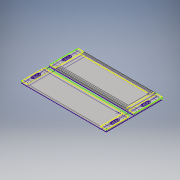
# Autodesk Inventor part: Fixture Base
Saved by Autodesk Inventor 2016 (Build 200138000, 138)
## iProperties
Created: 2016-04-07
Part Number: Fixture Base
Material: Generic
Document SubType Name: Modeling
Designer: Sam Clay
Density: 1 g/cm^3
Appearance: Default
Author: Sam Clay
Autodesk Inventor part; units mm, degrees
ref_plane "YZ Plane" through (0, 0, 0) normal (1, 0, 0) x (0, 1, 0)
ref_plane "XZ Plane" through (0, 0, 0) normal (0, 1, 0) x (-1, 0, 0)
ref_plane "XY Plane" through (0, 0, 0) normal (0, 0, 1) x (1, 0, 0)
sketch "Base Sketch" plane through (0, 0, 0) normal (0, 1, 0) x (-1, 0, 0)
  line L0 (0, 0) -> (660.4, 0)
  line L1 (660.4, 0) -> (660.4, 254)
  line L2 (660.4, 508) -> (0, 508)
  line L3 (0, 508) -> (0, 304.8)
  line L4 (0, 508) -> (-50.8, 508)
  line L5 (-50.8, 508) -> (-50.8, 304.8)
  line L6 (-50.8, 0) -> (0, 0)
  line L7 (0, 0) -> (0, 254)
  line L8 (660.4, 508) -> (711.2, 508)
  line L9 (711.2, 508) -> (711.2, 304.8)
  line L10 (711.2, 0) -> (660.4, 0)
  line L11 (660.4, 0) -> (660.4, 254)
  line L12 (660.4, 254) -> (660.4, 304.8)
  line L13 (711.2, 254) -> (711.2, 0)
  line L14 (0, 254) -> (0, 254)
  line L15 (-50.8, 254) -> (-50.8, 0)
  line L16 (711.2, 254) -> (660.4, 254)
  line L17 (711.2, 304.8) -> (660.4, 304.8)
  line L18 (711.2, 304.8) -> (711.2, 254)
  line L19 (711.2, 254) -> (711.2, 254)
  line L20 (660.4, 254) -> (660.4, 304.8)
  line L21 (660.4, 304.8) -> (660.4, 508)
  line L22 (0, 304.8) -> (0, 254)
  line L23 (0, 254) -> (0, 304.8)
  line L24 (-50.8, 254) -> (-50.8, 254)
  line L25 (-50.8, 304.8) -> (-50.8, 254)
  line L26 (660.4, 254) -> (0, 254)
  line L27 (660.4, 304.8) -> (0, 304.8)
  line L28 (0, 304.8) -> (-50.8, 304.8)
  line L29 (0, 254) -> (-50.8, 254)
  line L30 (0, 304.8) -> (0, 508)
  line L31 (0, 254) -> (0, 0)
  line L32 (660.4, 254) -> (660.4, 304.8)
  line L33 (660.4, 304.8) -> (660.4, 508)
  line L34 (635, 0) -> (635, 254)
  line L35 (25.4, 0) -> (25.4, 254)
  point P0 (660.4, 304.8)
  point P1 (660.4, 254)
  point P2 (660.4, 304.8)
  dimension "d0" = 660.4
  dimension "d87" = 50.8
  dimension "d88" = 50.8
  dimension "d165" = 254
  dimension "d166" = 50.8
  dimension "d167" = 203.2
  dimension "d172" = 25.4
  dimension "d173" = 25.4
  constraints: 72 end point, 43 parallel, 32 perpendicular, 14 coincident, 9 point on line, 3 horizontal
  measures "d0" distance of L2.end L2.start
  measures "d87" distance of L6.end L6.start
  measures "d88" distance of L10.start L10.end
  measures "d165" distance between parallel lines of L16 L0
  measures "d166" distance between parallel lines of L16 L17
  measures "d167" distance between parallel lines of L2 L17
  measures "d172" distance between parallel lines of L34 L1
  measures "d173" distance between parallel lines of L31 L35
extrude "Lower Level" add sketch "Base Sketch" along normal blind 17.78 contours L6 L15 L29 L7 | L28 L5 L4 L3 | L1 L16 L13 L10 | L21 L8 L9 L17
extrude "Base" add sketch "Base Sketch" along normal blind 19.05 contours L7 L26 L35 L0 | L35 L26 L34 L0 | L34 L26 L1 L0 | L3 L2 L21 L27
sketch "Tracks Sketch" plane through (0, 19.05, 0) normal (0, 1, 0) x (1, 0, 0)
  line L0 (-660.4, 0) -> (-660.4, -254) projected
  line L1 (0, -254) -> (0, 0) projected
  line L2 (-660.4, -22.987) -> (0, -22.987)
  line L3 (-660.4, -3.175) -> (0, -3.175)
  line L4 (-660.4, -231.013) -> (0, -231.013)
  line L5 (-660.4, -250.825) -> (0, -250.825)
  line L6 (-38.1, -35.687) -> (-660.4, -35.687)
  line L7 (-660.4, -35.687) -> (-660.4, -218.313)
  line L8 (-660.4, -218.313) -> (-38.1, -218.313)
  line L9 (-38.1, -218.313) -> (-38.1, -35.687)
  circle A0 centre (-41.91, -39.497) radius 8.89
  line L10 (-711.2, 0) -> (-711.2, -254) projected
  line L11 (50.8, -508) -> (50.8, -304.8) projected
  line L12 (-711.2, -508) -> (50.8, -508) projected
  line L13 (50.8, -304.8) -> (-711.2, -304.8) projected
  line L14 (-711.2, -254) -> (50.8, -254) projected
  line L15 (50.8, 0) -> (-711.2, 0) projected
  line L16 (-711.2, -304.8) -> (-711.2, -508) projected
  line L17 (50.8, -254) -> (50.8, 0) projected
  dimension "d170" = 19.812
  dimension "d171" = 19.812
  dimension "d174" = 38.1
  dimension "d175" = 12.7
  dimension "d176" = 12.7
  dimension "d177" = 182.626
  dimension "d178" = 17.78
  dimension "d179" = 5.08
  dimension "d180" = 5.08
  constraints: 16 end point, 9 point on line, 5 perpendicular, 2 parallel, 1 centre point, 1 horizontal
  measures "d170" distance between parallel lines of L5 L4
  measures "d171" distance between parallel lines of L2 L3
  measures "d174" distance between parallel lines of L1 L9
  measures "d175" distance between parallel lines of L2 L6
  measures "d176" distance between parallel lines of L4 L8
  measures "d177" distance between parallel lines of L8 L6
  measures "d178" diameter of A0
  measures "d179" distance edge to line of A0 L6
  measures "d180" distance edge to line of A0 L9
extrude "Pocket side" cut sketch "Tracks Sketch" against normal blind 3.175 contours L6 A0 L9 L8 L0 | A0 L9 L6 | L6 L9 A0
extrude "Tracks" cut sketch "Tracks Sketch" against normal blind 9.8425 contours L3 L1 L2 L0 | L1 L5 L0 L4
extrude "Interior Tracks" [suppressed]
sketch "Handle Sketch" plane through (0, 17.78, 0) normal (0, 1, 0) x (1, 0, 0)
  line L0 (-711.2, -254) -> (-660.4, -254) projected
  line L1 (-660.4, -254) -> (-660.4, -250.825) projected
  line L2 (-660.4, -250.825) -> (-660.4, -231.013) projected
  line L3 (-660.4, -231.013) -> (-660.4, -218.313) projected
  line L4 (-660.4, -218.313) -> (-660.4, -35.687) projected
  line L5 (-660.4, -35.687) -> (-660.4, -22.987) projected
  line L6 (-660.4, -22.987) -> (-660.4, -3.175) projected
  line L7 (-660.4, -3.175) -> (-660.4, 0) projected
  line L8 (-660.4, 0) -> (-711.2, 0) projected
  line L9 (-711.2, 0) -> (-711.2, -254) projected
  line L10 (50.8, 0) -> (0, 0) projected
  line L11 (0, 0) -> (0, -3.175) projected
  line L12 (0, -3.175) -> (0, -22.987) projected
  line L13 (0, -22.987) -> (0, -231.013) projected
  line L14 (0, -231.013) -> (0, -250.825) projected
  line L15 (0, -250.825) -> (0, -254) projected
  line L16 (0, -254) -> (50.8, -254) projected
  line L17 (50.8, -254) -> (50.8, 0) projected
  line L18 (0, -508) -> (50.8, -508) projected
  line L19 (50.8, -508) -> (50.8, -304.8) projected
  line L20 (50.8, -304.8) -> (0, -304.8) projected
  line L21 (0, -304.8) -> (0, -508) projected
  line L22 (-660.4, -508) -> (-660.4, -304.8) projected
  line L23 (-660.4, -304.8) -> (-711.2, -304.8) projected
  line L24 (-711.2, -304.8) -> (-711.2, -508) projected
  line L25 (-711.2, -508) -> (-660.4, -508) projected
  line L26 (-660.4, 0) -> (-711.2, 0) construction
  line L27 (-685.8, 0) -> (-685.8, -508) construction
  line L28 (25.4, 0) -> (25.4, -508) construction
  line L29 (-685.8, -88.9) -> (-685.8, -165.1) construction
  line L30 (-698.5, -101.6) -> (-698.5, -152.4)
  line L31 (-673.1, -152.4) -> (-673.1, -101.6)
  arc A0 (-673.1, -101.6) -> (-698.5, -101.6) centre (-685.8, -101.6) ccw
  arc A1 (-698.5, -152.4) -> (-673.1, -152.4) centre (-685.8, -152.4) ccw
  line L32 (25.4, -88.9) -> (25.4, -165.1) construction
  line L33 (12.7, -101.6) -> (12.7, -152.4)
  line L34 (38.1, -152.4) -> (38.1, -101.6)
  arc A2 (38.1, -101.6) -> (12.7, -101.6) centre (25.4, -101.6) ccw
  arc A3 (12.7, -152.4) -> (38.1, -152.4) centre (25.4, -152.4) ccw
  line L35 (-685.8, -368.3) -> (-685.8, -444.5) construction
  line L36 (-698.5, -381) -> (-698.5, -431.8)
  line L37 (-673.1, -431.8) -> (-673.1, -381)
  arc A4 (-673.1, -381) -> (-698.5, -381) centre (-685.8, -381) ccw
  arc A5 (-698.5, -431.8) -> (-673.1, -431.8) centre (-685.8, -431.8) ccw
  line L38 (25.4, -368.3) -> (25.4, -444.5) construction
  line L39 (12.7, -381) -> (12.7, -431.8)
  line L40 (38.1, -431.8) -> (38.1, -381)
  arc A6 (38.1, -381) -> (12.7, -381) centre (25.4, -381) ccw
  arc A7 (12.7, -431.8) -> (38.1, -431.8) centre (25.4, -431.8) ccw
  point P0 (-685.8, -25.4)
  point P1 (-685.8, -50.8)
  point P2 (-685.8, -203.2)
  point P3 (-685.8, -228.6)
  point P4 (-685.8, -317.5)
  point P5 (-685.8, -342.9)
  point P6 (-685.8, -469.9)
  point P7 (-685.8, -495.3)
  point P8 (25.4, -495.3)
  point P9 (25.4, -469.9)
  point P10 (25.4, -342.9)
  point P11 (25.4, -317.5)
  point P12 (25.4, -228.6)
  point P13 (25.4, -203.2)
  point P14 (25.4, -50.8)
  point P15 (25.4, -25.4)
  point P16 (-685.8, -127)
  point P17 (25.4, -127)
  point P18 (-685.8, -406.4)
  point P19 (25.4, -406.4)
  dimension "d181" = 25.4
  dimension "d182" = 25.4
  dimension "d183" = 25.4
  dimension "d184" = 25.4
  dimension "d185" = 25.4
  dimension "d186" = 25.4
  dimension "d187" = 25.4
  dimension "d188" = 25.4
  dimension "d189" = 25.4
  dimension "d190" = 25.4
  dimension "d191" = 12.7
  dimension "d192" = 25.4
  dimension "d193" = 12.7
  dimension "d194" = 25.4
  dimension "d195" = 12.7
  dimension "d196" = 25.4
  dimension "d197" = 12.7
  dimension "d198" = 25.4
  dimension "d199" = 76.2
  dimension "d200" = 25.4
  dimension "d201" = 127
  dimension "d202" = 76.2
  dimension "d203" = 25.4
  dimension "d204" = 127
  dimension "d205" = 76.2
  dimension "d206" = 25.4
  dimension "d207" = 76.2
  dimension "d208" = 25.4
  dimension "d209" = 101.6
  dimension "d210" = 101.6
  constraints: 32 end point, 24 point on circle, 16 tangent, 8 centre point, 8 midpoint, 8 point on line, 4 parallel, 2 horizontal, 30 other
  measures "d183" distance from line of point (-685.8, -25.4) L8
  measures "d184" distance of point (-685.8, -25.4) point (-685.8, -50.8)
  measures "d185" distance from line of L0 point (-685.8, -228.6)
  measures "d186" distance of point (-685.8, -203.2) point (-685.8, -228.6)
  measures "d187" distance from line of point (25.4, -25.4) L10
  measures "d188" distance of point (25.4, -50.8) point (25.4, -25.4)
  measures "d189" distance from line of L16 point (25.4, -228.6)
  measures "d190" distance of point (25.4, -203.2) point (25.4, -228.6)
  measures "d191" distance from line of point (-685.8, -317.5) L23
  measures "d192" distance of point (-685.8, -342.9) point (-685.8, -317.5)
  measures "d193" distance from line of L25 point (-685.8, -495.3)
  measures "d194" distance of point (-685.8, -469.9) point (-685.8, -495.3)
  measures "d195" distance from line of L18 point (25.4, -495.3)
  measures "d196" distance of point (25.4, -469.9) point (25.4, -495.3)
  measures "d197" distance from line of point (25.4, -317.5) L20
  measures "d198" distance of point (25.4, -342.9) point (25.4, -317.5)
  measures "d199" distance of L29.start L29.end
  measures "d200" diameter of A1
  measures "d201" distance from line of L8 point (-685.8, -127)
  measures "d202" distance of L32.start L32.end
  measures "d203" diameter of A3
  measures "d204" distance from line of L10 point (25.4, -127)
  measures "d205" distance of L35.start L35.end
  measures "d206" diameter of A5
  measures "d207" distance of L38.start L38.end
  measures "d208" diameter of A7
  measures "d209" distance from line of point (-685.8, -406.4) L23
  measures "d210" distance from line of point (25.4, -406.4) L20
sketch "Origin Sketch" plane through (0, 19.05, 0) normal (0, 1, 0) x (1, 0, 0)
  line L0 (0, -290.449) -> (-660.4, -290.449)
  line L1 (-660.4, -290.449) -> (-711.2, -290.449)
  line L2 (-711.2, 0) -> (-711.2, -254)
  line L3 (0, -290.449) -> (50.8, -290.449)
  line L4 (50.8, -254) -> (50.8, 0)
  line L5 (-660.4, -35.687) -> (-49.9422, -35.687) projected
  line L6 (-25.4, 0) -> (-25.4, -254) projected
  line L7 (0, -304.8) -> (-660.4, -304.8) projected
  line L8 (0, -304.8) -> (0, -508) projected
  point P0 (0, 0)
  point P1 (-25.4, -35.687)
  point P2 (-711.2, -508)
  point P3 (50.8, -508)
  point P4 (-25.4, -317.5)
  dimension "d211" = 12.7
  dimension "d212" = 25.4
  constraints: 10 end point, 5 point on line, 1 horizontal
  measures "d211" distance from line of L7 point (-25.4, -317.5)
  measures "d212" distance from line of L8 point (-25.4, -317.5)
extrude "Handles" cut sketch "Handle Sketch" against normal through all contours A0 L31 A1 L30 | A2 L34 A3 L33 | A4 L37 A5 L36 | A6 L40 A7 L39
body "Solid1"
